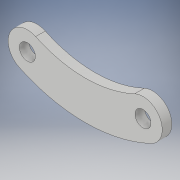
# Autodesk Inventor part: linkageA
Saved by Autodesk Inventor 2017 (Build 210142000, 142)
## iProperties
Created: 2016-08-20
Part Number: linkageA
Material: Generic
Document SubType Name: Modeling
Designer: Nic
Density: 1 g/cm^3
Appearance: Default
Author: Nic
Autodesk Inventor part; units mm, degrees
ref_plane "YZ Plane" through (0, 0, 0) normal (1, 0, 0) x (0, 1, 0)
ref_plane "XZ Plane" through (0, 0, 0) normal (0, 1, 0) x (-1, 0, 0)
ref_plane "XY Plane" through (0, 0, 0) normal (0, 0, 1) x (1, 0, 0)
sketch "Sketch1" plane through (0, 0, 0) normal (0, 0, 1) x (1, 0, 0)
  circle A0 centre (0, 0) radius 1.25
  line L0 (0, 0) -> (18, 0) construction
  circle A1 centre (18, 0) radius 1.25
  arc A2 (1.2857, 2.7105) -> (-1.2857, -2.7105) centre (0, 0) ccw
  arc A3 (19.2857, -2.7105) -> (16.7143, 2.7105) centre (18, 0) ccw
  arc A4 (1.2857, 2.7105) -> (16.7143, 2.7105) centre (9, 18.9737) ccw
  arc A5 (-1.2857, -2.7105) -> (19.2857, -2.7105) centre (9, 18.9737) ccw
  dimension "d0" = 2.5
  dimension "d1" = 18
  dimension "d8" = 6
  dimension "d17" = 18
  constraints: 8 point on circle, 6 centre point, 5 coincident, 3 tangent, 2 end point, 2 equal radius, 1 horizontal
  measures "d0" diameter of A0
  measures "d1" distance of L0.start L0.end
  measures "d8" diameter of A2
  measures "d17" radius of A4
extrude "Extrusion1" add sketch "Sketch1" along normal blind 1.5
body "Solid1"
